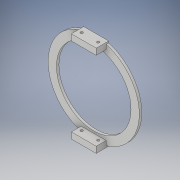
# Autodesk Inventor part: LED_Ring
Saved by Autodesk Inventor 2017 (Build 210142000, 142)
## iProperties
Part Number: LED_Ring
Material: Generisch
Document SubType Name: Modeling
Designer: Fabio
Density: 1 g/cm^3
Appearance: Vorgabe
Author: Fabio
Autodesk Inventor part; units mm, degrees
ref_plane "YZ Plane" through (0, 0, 0) normal (1, 0, 0) x (0, 1, 0)
ref_plane "XZ Plane" through (0, 0, 0) normal (0, 1, 0) x (-1, 0, 0)
ref_plane "XY Plane" through (0, 0, 0) normal (0, 0, 1) x (1, 0, 0)
sketch "Skizze1" plane through (0, 0, 0) normal (0, 1, 0) x (-1, 0, 0)
  circle A0 centre (0, 0) radius 55
  circle A1 centre (0, 0) radius 45
  dimension "d0" = 110
  dimension "d1" = 90
  constraints: 2 centre point, 2 coincident
  measures "d0" diameter of A0
  measures "d1" diameter of A1
extrude "Extrusion1" add sketch "Skizze1" along normal blind 3
sketch "Skizze2" plane through (0, 3, 0) normal (0, 1, 0) x (1, 0, 0)
  line L0 (15, -55) -> (-15, -55)
  line L1 (-15, -55) -> (-15, -47.5)
  line L2 (-15, -47.5) -> (15, -47.5)
  line L3 (15, -47.5) -> (15, -55)
  line L4 (15, -55) -> (-15, -47.5) construction
  line L5 (-15, -55) -> (15, -47.5) construction
  line L6 (0, 0) -> (0, -51.25) construction
  line L7 (-15, 55) -> (15, 55)
  line L8 (15, 55) -> (15, 47.5)
  line L9 (15, 47.5) -> (-15, 47.5)
  line L10 (-15, 47.5) -> (-15, 55)
  line L11 (-15, 55) -> (15, 47.5) construction
  line L12 (15, 55) -> (-15, 47.5) construction
  circle A0 centre (0, 0) radius 55 projected
  point P0 (0, 51.25)
  dimension "d4" = 30
  dimension "d12" = 360
  dimension "d14" = 47.5
  constraints: 26 end point, 4 midpoint, 2 parallel, 1 horizontal, 1 perpendicular, 1 tangent, 1 vertical, 23 other
  measures "d4" distance of L1.end L2.end
  measures "d14" distance from line of point (0, 0) L2
extrude "Extrusion2" add sketch "Skizze2" against normal blind 15 contours L0 A0 L3 | L0 L1 A0 | A0 L1 L2 L3 | A0 L8 L9 L10 | L10 L7 A0 | A0 L7 L8
sketch "Skizze3" plane through (15, 3, -55) normal (0, 0, -1) x (-1, 0, 0)
  line L0 (15, -3) -> (15, -21.7496) construction
  line L1 (30, 0) -> (30, -15) construction
  line L2 (30, -7.5) -> (0, -7.5) construction
  line L3 (0, 0) -> (0, -15) construction
  point P0 (5, -7.5)
  point P1 (25, -7.5)
  dimension "d19" = 20
  dimension "d20" = 10
  constraints: 4 end point, 2 midpoint, 2 point on line, 1 vertical
  measures "d19" distance of point (25, -7.5) point (5, -7.5)
  measures "d20" distance from line of point (5, -7.5) L0
hole "Bohrung1" at (10, -4.5, -55) at (-10, -4.5, -55) direction (0, 0, 1) diameter 3 end through all
